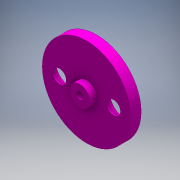
# Autodesk Inventor part: magnet_holder
Saved by Autodesk Inventor 2016 (Build 200138000, 138)
## iProperties
Created: 2016-04-25
Part Number: magnet_holder
Material: Plastique ABS
Document SubType Name: Modeling
Designer: tmonglon
Density: 1.06 g/cm^3
Appearance: Magenta
Mass: 1.46981 g
Surface Area: 14.8564 cm^2
Volume: 1.38661 cm^3
Author: tmonglon
Autodesk Inventor part; units mm, degrees
ref_plane "YZ Plane" through (0, 0, 0) normal (1, 0, 0) x (0, 1, 0)
ref_plane "XZ Plane" through (0, 0, 0) normal (0, 1, 0) x (-1, 0, 0)
ref_plane "XY Plane" through (0, 0, 0) normal (0, 0, 1) x (1, 0, 0)
sketch "Esquisse1" plane through (0, 0, 0) normal (0, 0, 1) x (1, 0, 0)
  line L0 (0, 0) -> (-13, 0)
  line L1 (-13, 0) -> (-13, 3)
  line L2 (-13, 3) -> (0, 3)
  line L3 (0, 3) -> (0, 0)
  line L4 (0, 3) -> (-6, 3)
  line L5 (0, 2.3367) -> (0, 3)
  line L6 (0, 0) -> (-3, 0)
  line L7 (-3, 0) -> (-3, -2)
  line L8 (-3, -2) -> (0, -2)
  line L9 (0, -2) -> (0, 0)
  line L10 (-2.2236, 3) -> (-3.9121, 3)
  line L11 (0, 3) -> (-3, 3)
  line L12 (-3, 3) -> (-3, 4)
  line L13 (-3, 4) -> (0, 4)
  line L14 (0, 4) -> (0, 3)
  line L15 (-1.05, 4) -> (-1.05, -2)
  line L16 (-4, 3) -> (-12, 3)
  line L17 (-12, 3) -> (-12, 0.5)
  line L18 (-12, 0.5) -> (-4, 0.5)
  line L19 (-4, 0.5) -> (-4, 3)
  dimension "d0" = 2
  dimension "d1" = 13
  dimension "d2" = 3
  dimension "d4" = 3
  dimension "d5" = 3
  dimension "d6" = 1
  dimension "d7" = 6
  dimension "d8" = 1.05
  dimension "d9" = 2.5
  dimension "d10" = 8
  dimension "d11" = 1
  constraints: 40 end point, 8 parallel, 6 horizontal, 5 perpendicular, 4 point on line
  measures "d0" distance of L6.end L7.end
  measures "d1" distance of L1.end L2.end
  measures "d2" distance of L7.end L8.end
  measures "d4" distance of L0.end L1.end
  measures "d5" distance of L12.end L13.end
  measures "d6" distance of L11.end L12.end
  measures "d7" distance between parallel lines of L8 L13
  measures "d8" distance between parallel lines of L3 L15
  measures "d9" distance of L16.end L17.end
  measures "d10" distance of L17.end L18.end
  measures "d11" distance between parallel lines of L1 L17
revolve "Révolution1" add sketch "Esquisse1" angle 360 about axis through (0, 4, 0) along (0, -1, 0)
hole "Perçage1" at (0, 4, 0) direction (0, -1, 0) diameter 2.1 end through all
sketch "Esquisse2" plane through (0, 3, 0) normal (0, 1, 0) x (1, 0, 0)
  circle A0 centre (-7.95, 0) radius 4.05
  circle A1 centre (7.95, 0) radius 4.05
  circle A2 centre (-7.95, 0) radius 2
  circle A3 centre (7.95, 0) radius 2
  point P0 (0, 0)
  dimension "d22" = 8.1
  dimension "d23" = 8.1
  dimension "d25" = 7.95
  dimension "d26" = 7.95
  dimension "d29" = 4
  dimension "d30" = 4
  constraints: 4 centre point, 2 coincident
  measures "d22" diameter of A0
  measures "d23" diameter of A1
  measures "d25" distance of point (0, 0) A0.centre
  measures "d26" distance of A1.centre point (0, 0)
  measures "d29" diameter of A2
  measures "d30" diameter of A3
extrude "Extrusion1" cut sketch "Esquisse2" against normal blind 2.5 contours A0 | A1 | A2 | A3
extrude "Extrusion2" cut sketch "Esquisse2" against normal through all contours A2 | A3
